Autodesk Inventor part; units mm, degrees
(part 3 of 4)
  spline S550 degree 2 poles (-51.993, -43.6703) (-51.7908, -43.577) (-51.241, -43.5069) (-50.922, -43.4888) knots 0 0 0 1 2 2 2
  line L465 (-50.922, -43.4888) -> (-50.922, -43.411)
  spline S551 degree 2 poles (-50.922, -43.411) (-50.922, -43.271) (-51.0076, -43.0972) (-51.0854, -43.0479) knots 0 0 0 1 2 2 2
  spline S552 degree 2 poles (-51.0854, -43.0479) (-51.1632, -42.9987) (-51.3862, -42.9676) (-51.5055, -42.9676) knots 0 0 0 1 2 2 2
  spline S553 degree 2 poles (-51.5055, -42.9676) (-51.6455, -42.9676) (-52.0241, -43.0505) (-52.2135, -43.1309) knots 0 0 0 1 2 2 2
  line L466 (-52.2135, -43.1309) -> (-52.2368, -43.1309)
  line L467 (-52.2368, -43.1309) -> (-52.2368, -42.7186)
  spline S554 degree 2 poles (-52.2368, -42.7186) (-52.1253, -42.6875) (-51.7078, -42.6097) (-51.5029, -42.6097) knots 0 0 0 1 2 2 2
  spline S555 degree 2 poles (-51.5029, -42.6097) (-51.254, -42.6097) (-50.9143, -42.6875) (-50.7794, -42.7886) knots 0 0 0 1 2 2 2
  spline S556 degree 2 poles (-50.7794, -42.7886) (-50.6472, -42.8872) (-50.5175, -43.2009) (-50.5175, -43.4266) knots 0 0 0 1 2 2 2
  line L468 (-50.5175, -43.4266) -> (-50.5175, -45.068)
  line L469 (-50.5175, -45.068) -> (-50.922, -45.068)
  line L470 (-50.922, -45.068) -> (-50.922, -44.8139)
  line L471 (-50.922, -44.4768) -> (-50.922, -43.8103)
  spline S557 degree 2 poles (-50.922, -43.8103) (-51.0673, -43.8233) (-51.5055, -43.8674) (-51.643, -43.9089) knots 0 0 0 1 2 2 2
  spline S558 degree 2 poles (-51.643, -43.9089) (-51.8037, -43.9582) (-52.0138, -44.163) (-52.0138, -44.3445) knots 0 0 0 1 2 2 2
  spline S559 degree 2 poles (-52.0138, -44.3445) (-52.0138, -44.552) (-51.7804, -44.762) (-51.5574, -44.762) knots 0 0 0 1 2 2 2
  spline S560 degree 2 poles (-51.5574, -44.762) (-51.3681, -44.762) (-51.0569, -44.5987) (-50.922, -44.4768) knots 0 0 0 1 2 2 2
  line L472 (-48.0643, -42.6667) -> (-49.3558, -45.9523)
  line L473 (-49.3558, -45.9523) -> (-49.7888, -45.9523)
  line L474 (-49.7888, -45.9523) -> (-49.3583, -44.9513)
  line L475 (-49.3583, -44.9513) -> (-50.2297, -42.6667)
  line L476 (-50.2297, -42.6667) -> (-49.794, -42.6667)
  line L477 (-49.794, -42.6667) -> (-49.1379, -44.4457)
  line L478 (-49.1379, -44.4457) -> (-48.4844, -42.6667)
  line L479 (-48.4844, -42.6667) -> (-48.0643, -42.6667)
  spline S561 degree 2 poles (-45.7849, -43.8674) (-45.7849, -44.4742) (-46.3684, -45.1355) (-46.8559, -45.1355) knots 0 0 0 1 2 2 2
  spline S562 degree 2 poles (-46.8559, -45.1355) (-47.3564, -45.1355) (-47.9295, -44.4535) (-47.9295, -43.8674) knots 0 0 0 1 2 2 2
  spline S563 degree 2 poles (-47.9295, -43.8674) (-47.9295, -43.2658) (-47.3383, -42.5993) (-46.8559, -42.5993) knots 0 0 0 1 2 2 2
  spline S564 degree 2 poles (-46.8559, -42.5993) (-46.3684, -42.5993) (-45.7849, -43.2632) (-45.7849, -43.8674) knots 0 0 0 1 2 2 2
  spline S565 degree 2 poles (-46.2024, -43.8674) (-46.2024, -43.4006) (-46.5421, -42.9468) (-46.8559, -42.9468) knots 0 0 0 1 2 2 2
  spline S566 degree 2 poles (-46.8559, -42.9468) (-47.1697, -42.9468) (-47.512, -43.4006) (-47.512, -43.8674) knots 0 0 0 1 2 2 2
  spline S567 degree 2 poles (-47.512, -43.8674) (-47.512, -44.3212) (-47.1697, -44.788) (-46.8559, -44.788) knots 0 0 0 1 2 2 2
  spline S568 degree 2 poles (-46.8559, -44.788) (-46.5447, -44.788) (-46.2024, -44.329) (-46.2024, -43.8674) knots 0 0 0 1 2 2 2
  line L480 (-42.4605, -42.6667) -> (-43.0699, -45.068)
  line L481 (-43.0699, -45.068) -> (-43.4433, -45.068)
  line L482 (-43.4433, -45.068) -> (-44.0293, -43.2165)
  line L483 (-44.0293, -43.2165) -> (-44.6128, -45.068)
  line L484 (-44.6128, -45.068) -> (-44.9836, -45.068)
  line L485 (-44.9836, -45.068) -> (-45.5982, -42.6667)
  line L486 (-45.5982, -42.6667) -> (-45.1781, -42.6667)
  line L487 (-45.1781, -42.6667) -> (-44.7528, -44.5261)
  line L488 (-44.7528, -44.5261) -> (-44.1849, -42.6667)
  line L489 (-44.1849, -42.6667) -> (-43.8504, -42.6667)
  line L490 (-43.8504, -42.6667) -> (-43.2669, -44.5261)
  line L491 (-43.2669, -44.5261) -> (-42.8676, -42.6667)
  line L492 (-42.8676, -42.6667) -> (-42.4605, -42.6667)
  spline S569 degree 2 poles (-40.7671, -44.8139) (-40.8164, -44.8502) (-40.9823, -44.9799) (-41.0601, -45.0188) knots 0 0 0 1 2 2 2
  spline S570 degree 2 poles (-41.0601, -45.0188) (-41.1665, -45.0758) (-41.3661, -45.1355) (-41.5477, -45.1355) knots 0 0 0 1 2 2 2
  spline S571 degree 2 poles (-41.5477, -45.1355) (-41.6955, -45.1355) (-41.9626, -45.024) (-42.0637, -44.9228) knots 0 0 0 1 2 2 2
  spline S572 degree 2 poles (-42.0637, -44.9228) (-42.1596, -44.8243) (-42.2763, -44.5338) (-42.2763, -44.3731) knots 0 0 0 1 2 2 2
  spline S573 degree 2 poles (-42.2763, -44.3731) (-42.2763, -44.1241) (-42.0663, -43.7714) (-41.8381, -43.6703) knots 0 0 0 1 2 2 2
  spline S574 degree 2 poles (-41.8381, -43.6703) (-41.6358, -43.577) (-41.0861, -43.5069) (-40.7671, -43.4888) knots 0 0 0 1 2 2 2
  line L493 (-40.7671, -43.4888) -> (-40.7671, -43.411)
  spline S575 degree 2 poles (-40.7671, -43.411) (-40.7671, -43.271) (-40.8527, -43.0972) (-40.9305, -43.0479) knots 0 0 0 1 2 2 2
  spline S576 degree 2 poles (-40.9305, -43.0479) (-41.0083, -42.9987) (-41.2313, -42.9676) (-41.3506, -42.9676) knots 0 0 0 1 2 2 2
  spline S577 degree 2 poles (-41.3506, -42.9676) (-41.4906, -42.9676) (-41.8692, -43.0505) (-42.0585, -43.1309) knots 0 0 0 1 2 2 2
  line L494 (-42.0585, -43.1309) -> (-42.0818, -43.1309)
  line L495 (-42.0818, -43.1309) -> (-42.0818, -42.7186)
  spline S578 degree 2 poles (-42.0818, -42.7186) (-41.9703, -42.6875) (-41.5528, -42.6097) (-41.348, -42.6097) knots 0 0 0 1 2 2 2
  spline S579 degree 2 poles (-41.348, -42.6097) (-41.099, -42.6097) (-40.7593, -42.6875) (-40.6245, -42.7886) knots 0 0 0 1 2 2 2
  spline S580 degree 2 poles (-40.6245, -42.7886) (-40.4922, -42.8872) (-40.3626, -43.2009) (-40.3626, -43.4266) knots 0 0 0 1 2 2 2
  line L496 (-40.3626, -43.4266) -> (-40.3626, -45.068)
  line L497 (-40.3626, -45.068) -> (-40.7671, -45.068)
  line L498 (-40.7671, -45.068) -> (-40.7671, -44.8139)
  line L499 (-40.7671, -44.4768) -> (-40.7671, -43.8103)
  spline S581 degree 2 poles (-40.7671, -43.8103) (-40.9123, -43.8233) (-41.3506, -43.8674) (-41.488, -43.9089) knots 0 0 0 1 2 2 2
  spline S582 degree 2 poles (-41.488, -43.9089) (-41.6488, -43.9582) (-41.8588, -44.163) (-41.8588, -44.3445) knots 0 0 0 1 2 2 2
  spline S583 degree 2 poles (-41.8588, -44.3445) (-41.8588, -44.552) (-41.6254, -44.762) (-41.4024, -44.762) knots 0 0 0 1 2 2 2
  spline S584 degree 2 poles (-41.4024, -44.762) (-41.2131, -44.762) (-40.9019, -44.5987) (-40.7671, -44.4768) knots 0 0 0 1 2 2 2
  spline S585 degree 2 poles (-95.7083, -4.693) (-95.7083, -4.8875) (-95.842, -5.2327) (-95.9757, -5.3543) knots 0 0 0 1 2 2 2
  spline S586 degree 2 poles (-95.9757, -5.3543) (-96.1264, -5.4904) (-96.5373, -5.6193) (-96.8047, -5.6193) knots 0 0 0 1 2 2 2
  spline S587 degree 2 poles (-96.8047, -5.6193) (-97.0041, -5.6193) (-97.3541, -5.5901) (-97.4878, -5.5609) knots 0 0 0 1 2 2 2
  line L500 (-97.4878, -5.5609) -> (-97.4878, -4.9531)
  line L501 (-97.4878, -4.9531) -> (-97.4198, -4.9531)
  spline S588 degree 2 poles (-97.4198, -4.9531) (-97.3298, -4.9896) (-97.1329, -5.0528) (-96.9773, -5.0528) knots 0 0 0 1 2 2 2
  spline S589 degree 2 poles (-96.9773, -5.0528) (-96.778, -5.0528) (-96.5616, -4.941) (-96.5178, -4.8389) knots 0 0 0 1 2 2 2
  spline S590 degree 2 poles (-96.5178, -4.8389) (-96.4716, -4.7392) (-96.4619, -4.4815) (-96.4619, -4.321) knots 0 0 0 1 2 2 2
  line L502 (-96.4619, -4.321) -> (-96.4619, -3.1176)
  line L503 (-96.4619, -3.1176) -> (-97.1475, -3.1176)
  line L504 (-97.1475, -3.1176) -> (-97.1475, -2.5731)
  line L505 (-97.1475, -2.5731) -> (-95.7083, -2.5731)
  line L506 (-95.7083, -2.5731) -> (-95.7083, -4.693)
  spline S591 degree 2 poles (-93.0024, -4.6638) (-93.0024, -4.8851) (-93.1653, -5.2473) (-93.3233, -5.3737) knots 0 0 0 1 2 2 2
  spline S592 degree 2 poles (-93.3233, -5.3737) (-93.4814, -5.5001) (-93.9117, -5.6363) (-94.2204, -5.6363) knots 0 0 0 1 2 2 2
  spline S593 degree 2 poles (-94.2204, -5.6363) (-94.5705, -5.6363) (-95.0713, -5.5196) (-95.2293, -5.4466) knots 0 0 0 1 2 2 2
  line L507 (-95.2293, -5.4466) -> (-95.2293, -4.7951)
  line L508 (-95.2293, -4.7951) -> (-95.1564, -4.7951)
  spline S594 degree 2 poles (-95.1564, -4.7951) (-94.9911, -4.8996) (-94.5462, -5.0552) (-94.3614, -5.0552) knots 0 0 0 1 2 2 2
  spline S595 degree 2 poles (-94.3614, -5.0552) (-94.252, -5.0552) (-93.9968, -5.0163) (-93.9092, -4.9531) knots 0 0 0 1 2 2 2
  spline S596 degree 2 poles (-93.9092, -4.9531) (-93.8412, -4.9021) (-93.7585, -4.7538) (-93.7585, -4.6201) knots 0 0 0 1 2 2 2
  spline S597 degree 2 poles (-93.7585, -4.6201) (-93.7585, -4.4864) (-93.8752, -4.3429) (-93.9724, -4.3089) knots 0 0 0 1 2 2 2
  spline S598 degree 2 poles (-93.9724, -4.3089) (-94.0697, -4.2749) (-94.3395, -4.2676) (-94.4441, -4.2676) knots 0 0 0 1 2 2 2
  line L509 (-94.4441, -4.2676) -> (-94.5729, -4.2676)
  line L510 (-94.5729, -4.2676) -> (-94.5729, -3.74)
  line L511 (-94.5729, -3.74) -> (-94.4538, -3.74)
  spline S599 degree 2 poles (-94.4538, -3.74) (-94.3177, -3.74) (-94.0867, -3.7157) (-94.0065, -3.6792) knots 0 0 0 1 2 2 2
  spline S600 degree 2 poles (-94.0065, -3.6792) (-93.9263, -3.6403) (-93.8363, -3.5042) (-93.8363, -3.3875) knots 0 0 0 1 2 2 2
  spline S601 degree 2 poles (-93.8363, -3.3875) (-93.8363, -3.2951) (-93.9214, -3.1808) (-93.9822, -3.1492) knots 0 0 0 1 2 2 2
  spline S602 degree 2 poles (-93.9822, -3.1492) (-94.0551, -3.1128) (-94.2496, -3.0885) (-94.3177, -3.0885) knots 0 0 0 1 2 2 2
  spline S603 degree 2 poles (-94.3177, -3.0885) (-94.4271, -3.0885) (-94.658, -3.1395) (-94.765, -3.1808) knots 0 0 0 1 2 2 2
  spline S604 degree 2 poles (-94.765, -3.1808) (-94.8501, -3.2125) (-95.0348, -3.3146) (-95.0786, -3.3413) knots 0 0 0 1 2 2 2
  line L512 (-95.0786, -3.3413) -> (-95.1418, -3.3413)
  line L513 (-95.1418, -3.3413) -> (-95.1418, -2.6995)
  spline S605 degree 2 poles (-95.1418, -2.6995) (-94.9862, -2.6338) (-94.4611, -2.5099) (-94.1864, -2.5099) knots 0 0 0 1 2 2 2
  spline S606 degree 2 poles (-94.1864, -2.5099) (-93.919, -2.5099) (-93.5251, -2.6022) (-93.3865, -2.6922) knots 0 0 0 1 2 2 2
  spline S607 degree 2 poles (-93.3865, -2.6922) (-93.2334, -2.787) (-93.0802, -3.0787) (-93.0802, -3.2611) knots 0 0 0 1 2 2 2
  spline S608 degree 2 poles (-93.0802, -3.2611) (-93.0802, -3.5188) (-93.3768, -3.9029) (-93.6199, -3.9588) knots 0 0 0 1 2 2 2
  line L514 (-93.6199, -3.9588) -> (-93.6199, -3.988)
  spline S609 degree 2 poles (-93.6199, -3.988) (-93.513, -4.0026) (-93.3088, -4.0804) (-93.2115, -4.1679) knots 0 0 0 1 2 2 2
  spline S610 degree 2 poles (-93.2115, -4.1679) (-93.1216, -4.2457) (-93.0024, -4.4937) (-93.0024, -4.6638) knots 0 0 0 1 2 2 2
  spline S611 degree 2 poles (-90.316, -4.552) (-90.316, -5.0261) (-90.9165, -5.6363) (-91.4417, -5.6363) knots 0 0 0 1 2 2 2
  spline S612 degree 2 poles (-91.4417, -5.6363) (-91.7042, -5.6363) (-92.1151, -5.4855) (-92.2585, -5.3372) knots 0 0 0 1 2 2 2
  spline S613 degree 2 poles (-92.2585, -5.3372) (-92.4287, -5.1646) (-92.611, -4.6176) (-92.611, -4.236) knots 0 0 0 1 2 2 2
  spline S614 degree 2 poles (-92.611, -4.236) (-92.611, -3.8421) (-92.4408, -3.2295) (-92.2488, -2.9937) knots 0 0 0 1 2 2 2
  spline S615 degree 2 poles (-92.2488, -2.9937) (-92.0665, -2.77) (-91.4733, -2.5172) (-91.0673, -2.5172) knots 0 0 0 1 2 2 2
  spline S616 degree 2 poles (-91.0673, -2.5172) (-90.919, -2.5172) (-90.6224, -2.5561) (-90.5689, -2.5682) knots 0 0 0 1 2 2 2
  line L515 (-90.5689, -2.5682) -> (-90.5689, -3.1565)
  line L516 (-90.5689, -3.1565) -> (-90.6224, -3.1565)
  spline S617 degree 2 poles (-90.6224, -3.1565) (-90.6759, -3.1298) (-90.919, -3.0642) (-91.0746, -3.0642) knots 0 0 0 1 2 2 2
  spline S618 degree 2 poles (-91.0746, -3.0642) (-91.4271, -3.0642) (-91.8112, -3.4361) (-91.8574, -3.7813) knots 0 0 0 1 2 2 2
  spline S619 degree 2 poles (-91.8574, -3.7813) (-91.7091, -3.6865) (-91.4052, -3.5747) (-91.2131, -3.5747) knots 0 0 0 1 2 2 2
  spline S620 degree 2 poles (-91.2131, -3.5747) (-91.0502, -3.5747) (-90.7658, -3.6622) (-90.6564, -3.7449) knots 0 0 0 1 2 2 2
  spline S621 degree 2 poles (-90.6564, -3.7449) (-90.5008, -3.864) (-90.316, -4.2505) (-90.316, -4.552) knots 0 0 0 1 2 2 2
  spline S622 degree 2 poles (-91.1937, -5.0042) (-91.1353, -4.9313) (-91.0721, -4.7611) (-91.0721, -4.5885) knots 0 0 0 1 2 2 2
  spline S623 degree 2 poles (-91.0721, -4.5885) (-91.0721, -4.4426) (-91.1451, -4.253) (-91.2107, -4.1971) knots 0 0 0 1 2 2 2
  spline S624 degree 2 poles (-91.2107, -4.1971) (-91.2788, -4.1387) (-91.4465, -4.0974) (-91.5413, -4.0974) knots 0 0 0 1 2 2 2
  spline S625 degree 2 poles (-91.5413, -4.0974) (-91.6216, -4.0974) (-91.7869, -4.1387) (-91.8598, -4.1679) knots 0 0 0 1 2 2 2
  spline S626 degree 2 poles (-91.8598, -4.1679) (-91.8598, -4.1873) (-91.8647, -4.2797) (-91.8647, -4.3502) knots 0 0 0 1 2 2 2
  spline S627 degree 2 poles (-91.8647, -4.3502) (-91.8647, -4.6103) (-91.7747, -4.924) (-91.7042, -5.0042) knots 0 0 0 1 2 2 2
  spline S628 degree 2 poles (-91.7042, -5.0042) (-91.6532, -5.0698) (-91.517, -5.1257) (-91.4441, -5.1257) knots 0 0 0 1 2 2 2
  spline S629 degree 2 poles (-91.4441, -5.1257) (-91.3833, -5.1257) (-91.2423, -5.065) (-91.1937, -5.0042) knots 0 0 0 1 2 2 2
  spline S630 degree 2 poles (-87.6783, -4.7392) (-87.6783, -4.9313) (-87.8387, -5.2643) (-87.9919, -5.3859) knots 0 0 0 1 2 2 2
  spline S631 degree 2 poles (-87.9919, -5.3859) (-88.1451, -5.5074) (-88.5851, -5.6436) (-88.8695, -5.6436) knots 0 0 0 1 2 2 2
  spline S632 degree 2 poles (-88.8695, -5.6436) (-89.1734, -5.6436) (-89.628, -5.505) (-89.7739, -5.3859) knots 0 0 0 1 2 2 2
  spline S633 degree 2 poles (-89.7739, -5.3859) (-89.9173, -5.2667) (-90.0535, -4.9434) (-90.0535, -4.7635) knots 0 0 0 1 2 2 2
  spline S634 degree 2 poles (-90.0535, -4.7635) (-90.0535, -4.5058) (-89.769, -4.163) (-89.4992, -4.0488) knots 0 0 0 1 2 2 2
  line L517 (-89.4992, -4.0488) -> (-89.4992, -4.0366)
  spline S635 degree 2 poles (-89.4992, -4.0366) (-89.7642, -3.9078) (-89.9733, -3.5407) (-89.9733, -3.3146) knots 0 0 0 1 2 2 2
  spline S636 degree 2 poles (-89.9733, -3.3146) (-89.9733, -3.1492) (-89.8274, -2.8599) (-89.684, -2.7457) knots 0 0 0 1 2 2 2
  spline S637 degree 2 poles (-89.684, -2.7457) (-89.5454, -2.6363) (-89.1248, -2.505) (-88.8622, -2.505) knots 0 0 0 1 2 2 2
  spline S638 degree 2 poles (-88.8622, -2.505) (-88.5851, -2.505) (-88.1718, -2.6241) (-88.0381, -2.7214) knots 0 0 0 1 2 2 2
  spline S639 degree 2 poles (-88.0381, -2.7214) (-87.9019, -2.8186) (-87.7561, -3.1006) (-87.7561, -3.2635) knots 0 0 0 1 2 2 2
  spline S640 degree 2 poles (-87.7561, -3.2635) (-87.7561, -3.4774) (-88.0041, -3.8202) (-88.2593, -3.9394) knots 0 0 0 1 2 2 2
  line L518 (-88.2593, -3.9394) -> (-88.2593, -3.9491)
  spline S641 degree 2 poles (-88.2593, -3.9491) (-87.9603, -4.0706) (-87.6783, -4.4645) (-87.6783, -4.7392) knots 0 0 0 1 2 2 2
  spline S642 degree 2 poles (-88.4222, -4.7708) (-88.4222, -4.6225) (-88.5486, -4.4669) (-88.7528, -4.3672) knots 0 0 0 1 2 2 2
  spline S643 degree 2 poles (-88.7528, -4.3672) (-88.8112, -4.3405) (-89.0324, -4.2554) (-89.1175, -4.2189) knots 0 0 0 1 2 2 2
  spline S644 degree 2 poles (-89.1175, -4.2189) (-89.1953, -4.2967) (-89.3193, -4.5301) (-89.3193, -4.6687) knots 0 0 0 1 2 2 2
  spline S645 degree 2 poles (-89.3193, -4.6687) (-89.3193, -4.8778) (-89.0519, -5.1282) (-88.8355, -5.1282) knots 0 0 0 1 2 2 2
  spline S646 degree 2 poles (-88.8355, -5.1282) (-88.7747, -5.1282) (-88.624, -5.0893) (-88.5656, -5.0504) knots 0 0 0 1 2 2 2
  spline S647 degree 2 poles (-88.5656, -5.0504) (-88.5, -5.0042) (-88.4222, -4.8778) (-88.4222, -4.7708) knots 0 0 0 1 2 2 2
  spline S648 degree 2 poles (-88.4878, -3.351) (-88.4878, -3.1979) (-88.6896, -3.0155) (-88.8622, -3.0155) knots 0 0 0 1 2 2 2
  spline S649 degree 2 poles (-88.8622, -3.0155) (-89.0276, -3.0155) (-89.2293, -3.1808) (-89.2293, -3.3024) knots 0 0 0 1 2 2 2
  spline S650 degree 2 poles (-89.2293, -3.3024) (-89.2293, -3.4215) (-89.1078, -3.5698) (-88.9789, -3.6306) knots 0 0 0 1 2 2 2
  spline S651 degree 2 poles (-88.9789, -3.6306) (-88.923, -3.6598) (-88.7674, -3.7206) (-88.6386, -3.7692) knots 0 0 0 1 2 2 2
  spline S652 degree 2 poles (-88.6386, -3.7692) (-88.5608, -3.6671) (-88.4878, -3.475) (-88.4878, -3.351) knots 0 0 0 1 2 2 2
  line L519 (-86.4457, -5.5731) -> (-87.158, -5.5731)
  line L520 (-87.158, -5.5731) -> (-87.158, -4.7805)
  line L521 (-87.158, -4.7805) -> (-86.4457, -4.7805)
  line L522 (-86.4457, -4.7805) -> (-86.4457, -5.5731)
  line L523 (-86.4457, -4.1022) -> (-87.158, -4.1022)
  line L524 (-87.158, -4.1022) -> (-87.158, -3.3097)
  line L525 (-87.158, -3.3097) -> (-86.4457, -3.3097)
  line L526 (-86.4457, -3.3097) -> (-86.4457, -4.1022)
  line L527 (-84.8582, -5.5731) -> (-83.8444, -2.5731)
  line L528 (-83.8444, -2.5731) -> (-83.0227, -2.5731)
  line L529 (-83.0227, -2.5731) -> (-82.0089, -5.5731)
  line L530 (-82.0089, -5.5731) -> (-82.7844, -5.5731)
  line L531 (-82.7844, -5.5731) -> (-82.9716, -4.9604)
  line L532 (-82.9716, -4.9604) -> (-83.9149, -4.9604)
  line L533 (-83.9149, -4.9604) -> (-84.1045, -5.5731)
  line L534 (-84.1045, -5.5731) -> (-84.8582, -5.5731)
  line L535 (-83.137, -4.4159) -> (-83.4433, -3.424)
  line L536 (-83.4433, -3.424) -> (-83.752, -4.4159)
  line L537 (-83.752, -4.4159) -> (-83.137, -4.4159)
  spline S653 degree 2 poles (-79.0332, -4.0755) (-79.0332, -4.4961) (-79.4003, -5.1573) (-79.6799, -5.3348) knots 0 0 0 1 2 2 2
  spline S654 degree 2 poles (-79.6799, -5.3348) (-79.9133, -5.4855) (-80.4627, -5.5731) (-80.7715, -5.5731) knots 0 0 0 1 2 2 2
  line L538 (-80.7715, -5.5731) -> (-81.7099, -5.5731)
  line L539 (-81.7099, -5.5731) -> (-81.7099, -2.5731)
  line L540 (-81.7099, -2.5731) -> (-80.7812, -2.5731)
  spline S655 degree 2 poles (-80.7812, -2.5731) (-80.4652, -2.5731) (-79.9133, -2.6533) (-79.6702, -2.8089) knots 0 0 0 1 2 2 2
  spline S656 degree 2 poles (-79.6702, -2.8089) (-79.376, -2.9985) (-79.0332, -3.6403) (-79.0332, -4.0755) knots 0 0 0 1 2 2 2
  spline S657 degree 2 poles (-79.8063, -4.0706) (-79.8063, -3.774) (-80.0105, -3.351) (-80.2196, -3.2319) knots 0 0 0 1 2 2 2
  spline S658 degree 2 poles (-80.2196, -3.2319) (-80.3728, -3.1492) (-80.7083, -3.1322) (-80.9417, -3.1322) knots 0 0 0 1 2 2 2
  line L541 (-80.9417, -3.1322) -> (-80.9562, -3.1322)
  line L542 (-80.9562, -3.1322) -> (-80.9562, -5.0115)
  line L543 (-80.9562, -5.0115) -> (-80.9417, -5.0115)
  spline S659 degree 2 poles (-80.9417, -5.0115) (-80.6888, -5.0115) (-80.3412, -4.9945) (-80.1831, -4.8948) knots 0 0 0 1 2 2 2
  spline S660 degree 2 poles (-80.1831, -4.8948) (-79.9984, -4.7781) (-79.8063, -4.3672) (-79.8063, -4.0706) knots 0 0 0 1 2 2 2
  line L544 (-76.0818, -2.5731) -> (-77.1126, -5.5731)
  line L545 (-77.1126, -5.5731) -> (-77.8979, -5.5731)
  line L546 (-77.8979, -5.5731) -> (-78.9287, -2.5731)
  line L547 (-78.9287, -2.5731) -> (-78.1483, -2.5731)
  line L548 (-78.1483, -2.5731) -> (-77.4943, -4.6079)
  line L549 (-77.4943, -4.6079) -> (-76.8428, -2.5731)
  line L550 (-76.8428, -2.5731) -> (-76.0818, -2.5731)
  line L551 (-76.1256, -5.5731) -> (-75.1118, -2.5731)
  line L552 (-75.1118, -2.5731) -> (-74.2901, -2.5731)
  line L553 (-74.2901, -2.5731) -> (-73.2763, -5.5731)
  line L554 (-73.2763, -5.5731) -> (-74.0519, -5.5731)
  line L555 (-74.0519, -5.5731) -> (-74.2391, -4.9604)
  line L556 (-74.2391, -4.9604) -> (-75.1823, -4.9604)
  line L557 (-75.1823, -4.9604) -> (-75.372, -5.5731)
  line L558 (-75.372, -5.5731) -> (-76.1256, -5.5731)
  line L559 (-74.4044, -4.4159) -> (-74.7107, -3.424)
  line L560 (-74.7107, -3.424) -> (-75.0194, -4.4159)
  line L561 (-75.0194, -4.4159) -> (-74.4044, -4.4159)
  line L562 (-70.4076, -5.5731) -> (-71.1321, -5.5731)
  line L563 (-71.1321, -5.5731) -> (-72.2893, -3.4823)
  line L564 (-72.2893, -3.4823) -> (-72.2893, -5.5731)
  line L565 (-72.2893, -5.5731) -> (-72.9773, -5.5731)
  line L566 (-72.9773, -5.5731) -> (-72.9773, -2.5731)
  line L567 (-72.9773, -2.5731) -> (-72.0535, -2.5731)
  line L568 (-72.0535, -2.5731) -> (-71.0956, -4.2919)
  line L569 (-71.0956, -4.2919) -> (-71.0956, -2.5731)
  line L570 (-71.0956, -2.5731) -> (-70.4076, -2.5731)
  line L571 (-70.4076, -2.5731) -> (-70.4076, -5.5731)
  spline S661 degree 2 poles (-68.5041, -5.6314) (-69.1799, -5.6314) (-69.9724, -4.8146) (-69.9724, -4.0755) knots 0 0 0 1 2 2 2
  spline S662 degree 2 poles (-69.9724, -4.0755) (-69.9724, -3.3632) (-69.1775, -2.5147) (-68.5016, -2.5147) knots 0 0 0 1 2 2 2
  spline S663 degree 2 poles (-68.5016, -2.5147) (-68.3241, -2.5147) (-68.0373, -2.5561) (-67.906, -2.5901) knots 0 0 0 1 2 2 2
  spline S664 degree 2 poles (-67.906, -2.5901) (-67.8039, -2.6217) (-67.5632, -2.7262) (-67.4878, -2.7651) knots 0 0 0 1 2 2 2
  line L572 (-67.4878, -2.7651) -> (-67.4878, -3.4799)
  line L573 (-67.4878, -3.4799) -> (-67.5632, -3.4799)
  spline S665 degree 2 poles (-67.5632, -3.4799) (-67.6191, -3.4313) (-67.7844, -3.2951) (-67.889, -3.2319) knots 0 0 0 1 2 2 2
  spline S666 degree 2 poles (-67.889, -3.2319) (-67.9935, -3.1663) (-68.2439, -3.0763) (-68.3825, -3.0763) knots 0 0 0 1 2 2 2
  spline S667 degree 2 poles (-68.3825, -3.0763) (-68.5454, -3.0763) (-68.8152, -3.1784) (-68.9392, -3.3073) knots 0 0 0 1 2 2 2
  spline S668 degree 2 poles (-68.9392, -3.3073) (-69.0511, -3.4215) (-69.1945, -3.8129) (-69.1945, -4.0779) knots 0 0 0 1 2 2 2
  spline S669 degree 2 poles (-69.1945, -4.0779) (-69.1945, -4.3575) (-69.0462, -4.7392) (-68.9246, -4.8559) knots 0 0 0 1 2 2 2
  spline S670 degree 2 poles (-68.9246, -4.8559) (-68.8079, -4.9702) (-68.5211, -5.0698) (-68.3776, -5.0698) knots 0 0 0 1 2 2 2
  spline S671 degree 2 poles (-68.3776, -5.0698) (-68.2293, -5.0698) (-67.9595, -4.9702) (-67.8671, -4.9094) knots 0 0 0 1 2 2 2
  spline S672 degree 2 poles (-67.8671, -4.9094) (-67.765, -4.8486) (-67.6118, -4.7197) (-67.5559, -4.6687) knots 0 0 0 1 2 2 2
  line L574 (-67.5559, -4.6687) -> (-67.4878, -4.6687)
  line L575 (-67.4878, -4.6687) -> (-67.4878, -5.3737)
  spline S673 degree 2 poles (-67.4878, -5.3737) (-67.5705, -5.4126) (-67.7869, -5.5099) (-67.9036, -5.5439) knots 0 0 0 1 2 2 2
  spline S674 degree 2 poles (-67.9036, -5.5439) (-68.0446, -5.5877) (-68.2901, -5.6314) (-68.5041, -5.6314) knots 0 0 0 1 2 2 2
  line L576 (-67.0429, -5.5731) -> (-67.0429, -2.5731)
  line L577 (-67.0429, -2.5731) -> (-65.0154, -2.5731)
  line L578 (-65.0154, -2.5731) -> (-65.0154, -3.1444)
  line L579 (-65.0154, -3.1444) -> (-66.2942, -3.1444)
  line L580 (-66.2942, -3.1444) -> (-66.2942, -3.6719)
  line L581 (-66.2942, -3.6719) -> (-65.1151, -3.6719)
  line L582 (-65.1151, -3.6719) -> (-65.1151, -4.2432)
  line L583 (-65.1151, -4.2432) -> (-66.2942, -4.2432)
  line L584 (-66.2942, -4.2432) -> (-66.2942, -5.0018)
  line L585 (-66.2942, -5.0018) -> (-65.0154, -5.0018)
  line L586 (-65.0154, -5.0018) -> (-65.0154, -5.5731)
  line L587 (-65.0154, -5.5731) -> (-67.0429, -5.5731)
  spline S675 degree 2 poles (-61.8282, -4.0755) (-61.8282, -4.4961) (-62.1953, -5.1573) (-62.4749, -5.3348) knots 0 0 0 1 2 2 2
  spline S676 degree 2 poles (-62.4749, -5.3348) (-62.7083, -5.4855) (-63.2577, -5.5731) (-63.5664, -5.5731) knots 0 0 0 1 2 2 2
  line L588 (-63.5664, -5.5731) -> (-64.5049, -5.5731)
  line L589 (-64.5049, -5.5731) -> (-64.5049, -2.5731)
  line L590 (-64.5049, -2.5731) -> (-63.5762, -2.5731)
  spline S677 degree 2 poles (-63.5762, -2.5731) (-63.2601, -2.5731) (-62.7083, -2.6533) (-62.4652, -2.8089) knots 0 0 0 1 2 2 2
  spline S678 degree 2 poles (-62.4652, -2.8089) (-62.171, -2.9985) (-61.8282, -3.6403) (-61.8282, -4.0755) knots 0 0 0 1 2 2 2
  spline S679 degree 2 poles (-62.6013, -4.0706) (-62.6013, -3.774) (-62.8055, -3.351) (-63.0146, -3.2319) knots 0 0 0 1 2 2 2
  spline S680 degree 2 poles (-63.0146, -3.2319) (-63.1677, -3.1492) (-63.5032, -3.1322) (-63.7366, -3.1322) knots 0 0 0 1 2 2 2
  line L591 (-63.7366, -3.1322) -> (-63.7512, -3.1322)
  line L592 (-63.7512, -3.1322) -> (-63.7512, -5.0115)
  line L593 (-63.7512, -5.0115) -> (-63.7366, -5.0115)
  spline S681 degree 2 poles (-63.7366, -5.0115) (-63.4838, -5.0115) (-63.1361, -4.9945) (-62.9781, -4.8948) knots 0 0 0 1 2 2 2
  spline S682 degree 2 poles (-62.9781, -4.8948) (-62.7934, -4.7781) (-62.6013, -4.3672) (-62.6013, -4.0706) knots 0 0 0 1 2 2 2
  spline S683 degree 2 poles (-57.4959, -4.0755) (-57.4959, -4.4961) (-57.863, -5.1573) (-58.1426, -5.3348) knots 0 0 0 1 2 2 2
  spline S684 degree 2 poles (-58.1426, -5.3348) (-58.376, -5.4855) (-58.9254, -5.5731) (-59.2342, -5.5731) knots 0 0 0 1 2 2 2
  line L594 (-59.2342, -5.5731) -> (-60.1726, -5.5731)
  line L595 (-60.1726, -5.5731) -> (-60.1726, -2.5731)
  line L596 (-60.1726, -2.5731) -> (-59.2439, -2.5731)
  spline S685 degree 2 poles (-59.2439, -2.5731) (-58.9279, -2.5731) (-58.376, -2.6533) (-58.1329, -2.8089) knots 0 0 0 1 2 2 2
  spline S686 degree 2 poles (-58.1329, -2.8089) (-57.8387, -2.9985) (-57.4959, -3.6403) (-57.4959, -4.0755) knots 0 0 0 1 2 2 2
  spline S687 degree 2 poles (-58.269, -4.0706) (-58.269, -3.774) (-58.4733, -3.351) (-58.6823, -3.2319) knots 0 0 0 1 2 2 2
  spline S688 degree 2 poles (-58.6823, -3.2319) (-58.8355, -3.1492) (-59.171, -3.1322) (-59.4044, -3.1322) knots 0 0 0 1 2 2 2
  line L597 (-59.4044, -3.1322) -> (-59.419, -3.1322)
  line L598 (-59.419, -3.1322) -> (-59.419, -5.0115)
  line L599 (-59.419, -5.0115) -> (-59.4044, -5.0115)
  spline S689 degree 2 poles (-59.4044, -5.0115) (-59.1515, -5.0115) (-58.8039, -4.9945) (-58.6459, -4.8948) knots 0 0 0 1 2 2 2
  spline S690 degree 2 poles (-58.6459, -4.8948) (-58.4611, -4.7781) (-58.269, -4.3672) (-58.269, -4.0706) knots 0 0 0 1 2 2 2
  line L600 (-55.5559, -5.5731) -> (-57.1702, -5.5731)
  line L601 (-57.1702, -5.5731) -> (-57.1702, -5.0504)
  line L602 (-57.1702, -5.0504) -> (-56.7399, -5.0504)
  line L603 (-56.7399, -5.0504) -> (-56.7399, -3.0958)
  line L604 (-56.7399, -3.0958) -> (-57.1702, -3.0958)
  line L605 (-57.1702, -3.0958) -> (-57.1702, -2.5731)
  line L606 (-57.1702, -2.5731) -> (-55.5559, -2.5731)
  line L607 (-55.5559, -2.5731) -> (-55.5559, -3.0958)
  line L608 (-55.5559, -3.0958) -> (-55.9862, -3.0958)
  line L609 (-55.9862, -3.0958) -> (-55.9862, -5.0504)
  line L610 (-55.9862, -5.0504) -> (-55.5559, -5.0504)
  line L611 (-55.5559, -5.0504) -> (-55.5559, -5.5731)
  spline S691 degree 2 poles (-52.748, -3.5188) (-52.748, -3.7278) (-52.8817, -4.1071) (-53.0057, -4.2335) knots 0 0 0 1 2 2 2
  spline S692 degree 2 poles (-53.0057, -4.2335) (-53.081, -4.3137) (-53.2658, -4.445) (-53.3752, -4.4912) knots 0 0 0 1 2 2 2
  spline S693 degree 2 poles (-53.3752, -4.4912) (-53.487, -4.5374) (-53.7472, -4.5909) (-53.9076, -4.5909) knots 0 0 0 1 2 2 2
  line L612 (-53.9076, -4.5909) -> (-54.3015, -4.5909)
  line L613 (-54.3015, -4.5909) -> (-54.3015, -5.5731)
  line L614 (-54.3015, -5.5731) -> (-55.0551, -5.5731)
  line L615 (-55.0551, -5.5731) -> (-55.0551, -2.5731)
  line L616 (-55.0551, -2.5731) -> (-53.8906, -2.5731)
  spline S694 degree 2 poles (-53.8906, -2.5731) (-53.6329, -2.5731) (-53.2561, -2.6679) (-53.1029, -2.77) knots 0 0 0 1 2 2 2
  spline S695 degree 2 poles (-53.1029, -2.77) (-52.9327, -2.8843) (-52.748, -3.2586) (-52.748, -3.5188) knots 0 0 0 1 2 2 2
  spline S696 degree 2 poles (-53.5211, -3.5382) (-53.5211, -3.4094) (-53.6426, -3.227) (-53.7253, -3.193) knots 0 0 0 1 2 2 2
  spline S697 degree 2 poles (-53.7253, -3.193) (-53.8323, -3.1468) (-54.0267, -3.1322) (-54.1945, -3.1322) knots 0 0 0 1 2 2 2
  line L617 (-54.1945, -3.1322) -> (-54.3015, -3.1322)
  line L618 (-54.3015, -3.1322) -> (-54.3015, -4.0317)
  line L619 (-54.3015, -4.0317) -> (-54.248, -4.0317)
  spline S698 degree 2 poles (-54.248, -4.0317) (-54.1434, -4.0317) (-53.9538, -4.0269) (-53.8833, -4.0147) knots 0 0 0 1 2 2 2
  spline S699 degree 2 poles (-53.8833, -4.0147) (-53.8225, -4.005) (-53.6888, -3.9466) (-53.6523, -3.9102) knots 0 0 0 1 2 2 2
  spline S700 degree 2 poles (-53.6523, -3.9102) (-53.5746, -3.8372) (-53.5211, -3.6744) (-53.5211, -3.5382) knots 0 0 0 1 2 2 2
  line L620 (-50.3436, -5.5731) -> (-52.3444, -5.5731)
  line L621 (-52.3444, -5.5731) -> (-52.3444, -2.5731)
  line L622 (-52.3444, -2.5731) -> (-51.5908, -2.5731)
  line L623 (-51.5908, -2.5731) -> (-51.5908, -5.0018)
  line L624 (-51.5908, -5.0018) -> (-50.3436, -5.0018)
  line L625 (-50.3436, -5.0018) -> (-50.3436, -5.5731)
  spline S701 degree 2 poles (-47.2536, -4.0731) (-47.2536, -4.8024) (-48.0316, -5.6363) (-48.7075, -5.6363) knots 0 0 0 1 2 2 2
  spline S702 degree 2 poles (-48.7075, -5.6363) (-49.3857, -5.6363) (-50.1588, -4.7927) (-50.1588, -4.0731) knots 0 0 0 1 2 2 2
  spline S703 degree 2 poles (-50.1588, -4.0731) (-50.1588, -3.351) (-49.3857, -2.5099) (-48.7075, -2.5099) knots 0 0 0 1 2 2 2
  spline S704 degree 2 poles (-48.7075, -2.5099) (-48.0316, -2.5099) (-47.2536, -3.3462) (-47.2536, -4.0731) knots 0 0 0 1 2 2 2
  spline S705 degree 2 poles (-48.0316, -4.0731) (-48.0316, -3.8032) (-48.141, -3.4264) (-48.2358, -3.3073) knots 0 0 0 1 2 2 2
  spline S706 degree 2 poles (-48.2358, -3.3073) (-48.3306, -3.1833) (-48.5737, -3.0763) (-48.705, -3.0763) knots 0 0 0 1 2 2 2
  spline S707 degree 2 poles (-48.705, -3.0763) (-48.8436, -3.0763) (-49.0697, -3.176) (-49.1742, -3.3024) knots 0 0 0 1 2 2 2
  spline S708 degree 2 poles (-49.1742, -3.3024) (-49.2666, -3.4191) (-49.3809, -3.8056) (-49.3809, -4.0731) knots 0 0 0 1 2 2 2
  spline S709 degree 2 poles (-49.3809, -4.0731) (-49.3809, -4.3502) (-49.2715, -4.7149) (-49.1767, -4.8389) knots 0 0 0 1 2 2 2
  spline S710 degree 2 poles (-49.1767, -4.8389) (-49.0818, -4.9629) (-48.8363, -5.0698) (-48.705, -5.0698) knots 0 0 0 1 2 2 2
  spline S711 degree 2 poles (-48.705, -5.0698) (-48.5713, -5.0698) (-48.3233, -4.9556) (-48.2334, -4.834) knots 0 0 0 1 2 2 2
  spline S712 degree 2 poles (-48.2334, -4.834) (-48.1361, -4.7027) (-48.0316, -4.3551) (-48.0316, -4.0731) knots 0 0 0 1 2 2 2
  line L626 (-43.7431, -5.5731) -> (-44.4919, -5.5731)
  line L627 (-44.4919, -5.5731) -> (-44.4919, -3.5844)
  line L628 (-44.4919, -3.5844) -> (-45.0365, -4.868)
  line L629 (-45.0365, -4.868) -> (-45.5519, -4.868)
  line L630 (-45.5519, -4.868) -> (-46.0964, -3.5844)
  line L631 (-46.0964, -3.5844) -> (-46.0964, -5.5731)
  line L632 (-46.0964, -5.5731) -> (-46.8063, -5.5731)
  line L633 (-46.8063, -5.5731) -> (-46.8063, -2.5731)
  line L634 (-46.8063, -2.5731) -> (-45.9384, -2.5731)
  line L635 (-45.9384, -2.5731) -> (-45.2723, -4.0536)
  line L636 (-45.2723, -4.0536) -> (-44.611, -2.5731)
  line L637 (-44.611, -2.5731) -> (-43.7431, -2.5731)
  line L638 (-43.7431, -2.5731) -> (-43.7431, -5.5731)
  line L639 (-43.4441, -5.5731) -> (-42.4303, -2.5731)
  line L640 (-42.4303, -2.5731) -> (-41.6086, -2.5731)
  line L641 (-41.6086, -2.5731) -> (-40.5948, -5.5731)
  line L642 (-40.5948, -5.5731) -> (-41.3703, -5.5731)
  line L643 (-41.3703, -5.5731) -> (-41.5575, -4.9604)
  line L644 (-41.5575, -4.9604) -> (-42.5008, -4.9604)
  line L645 (-42.5008, -4.9604) -> (-42.6904, -5.5731)
  line L646 (-42.6904, -5.5731) -> (-43.4441, -5.5731)
  line L647 (-41.7229, -4.4159) -> (-42.0292, -3.424)
  line L648 (-42.0292, -3.424) -> (-42.3379, -4.4159)
  line L649 (-42.3379, -4.4159) -> (-41.7229, -4.4159)
  spline S713 degree 2 poles (-36.3574, -4.0731) (-36.3574, -4.8024) (-37.1353, -5.6363) (-37.8112, -5.6363) knots 0 0 0 1 2 2 2
  spline S714 degree 2 poles (-37.8112, -5.6363) (-38.4895, -5.6363) (-39.2626, -4.7927) (-39.2626, -4.0731) knots 0 0 0 1 2 2 2
  spline S715 degree 2 poles (-39.2626, -4.0731) (-39.2626, -3.351) (-38.4895, -2.5099) (-37.8112, -2.5099) knots 0 0 0 1 2 2 2
  spline S716 degree 2 poles (-37.8112, -2.5099) (-37.1353, -2.5099) (-36.3574, -3.3462) (-36.3574, -4.0731) knots 0 0 0 1 2 2 2
  spline S717 degree 2 poles (-37.1353, -4.0731) (-37.1353, -3.8032) (-37.2447, -3.4264) (-37.3395, -3.3073) knots 0 0 0 1 2 2 2
  spline S718 degree 2 poles (-37.3395, -3.3073) (-37.4344, -3.1833) (-37.6775, -3.0763) (-37.8087, -3.0763) knots 0 0 0 1 2 2 2
  spline S719 degree 2 poles (-37.8087, -3.0763) (-37.9473, -3.0763) (-38.1734, -3.176) (-38.278, -3.3024) knots 0 0 0 1 2 2 2
  spline S720 degree 2 poles (-38.278, -3.3024) (-38.3703, -3.4191) (-38.4846, -3.8056) (-38.4846, -4.0731) knots 0 0 0 1 2 2 2
  spline S721 degree 2 poles (-38.4846, -4.0731) (-38.4846, -4.3502) (-38.3752, -4.7149) (-38.2804, -4.8389) knots 0 0 0 1 2 2 2
  spline S722 degree 2 poles (-38.2804, -4.8389) (-38.1856, -4.9629) (-37.94, -5.0698) (-37.8087, -5.0698) knots 0 0 0 1 2 2 2
  spline S723 degree 2 poles (-37.8087, -5.0698) (-37.675, -5.0698) (-37.4271, -4.9556) (-37.3371, -4.834) knots 0 0 0 1 2 2 2
  spline S724 degree 2 poles (-37.3371, -4.834) (-37.2399, -4.7027) (-37.1353, -4.3551) (-37.1353, -4.0731) knots 0 0 0 1 2 2 2
  line L650 (-33.9019, -3.1444) -> (-35.1613, -3.1444)
  line L651 (-35.1613, -3.1444) -> (-35.1613, -3.7108)
  line L652 (-35.1613, -3.7108) -> (-34.0016, -3.7108)
  line L653 (-34.0016, -3.7108) -> (-34.0016, -4.2821)
  line L654 (-34.0016, -4.2821) -> (-35.1613, -4.2821)
  line L655 (-35.1613, -4.2821) -> (-35.1613, -5.5731)
  line L656 (-35.1613, -5.5731) -> (-35.91, -5.5731)
  line L657 (-35.91, -5.5731) -> (-35.91, -2.5731)
  line L658 (-35.91, -2.5731) -> (-33.9019, -2.5731)
  line L659 (-33.9019, -2.5731) -> (-33.9019, -3.1444)
  line L660 (-32.3047, -5.5731) -> (-32.3047, -2.5731)
  line L661 (-32.3047, -2.5731) -> (-30.2771, -2.5731)
  line L662 (-30.2771, -2.5731) -> (-30.2771, -3.1444)
  line L663 (-30.2771, -3.1444) -> (-31.5559, -3.1444)
  line L664 (-31.5559, -3.1444) -> (-31.5559, -3.6719)
  line L665 (-31.5559, -3.6719) -> (-30.3768, -3.6719)
  line L666 (-30.3768, -3.6719) -> (-30.3768, -4.2432)
  line L667 (-30.3768, -4.2432) -> (-31.5559, -4.2432)
  line L668 (-31.5559, -4.2432) -> (-31.5559, -5.0018)
  line L669 (-31.5559, -5.0018) -> (-30.2771, -5.0018)
  line L670 (-30.2771, -5.0018) -> (-30.2771, -5.5731)
  line L671 (-30.2771, -5.5731) -> (-32.3047, -5.5731)
  line L672 (-27.1969, -5.5731) -> (-27.9214, -5.5731)
  line L673 (-27.9214, -5.5731) -> (-29.0786, -3.4823)
  line L674 (-29.0786, -3.4823) -> (-29.0786, -5.5731)
  line L675 (-29.0786, -5.5731) -> (-29.7666, -5.5731)
  line L676 (-29.7666, -5.5731) -> (-29.7666, -2.5731)
  line L677 (-29.7666, -2.5731) -> (-28.8428, -2.5731)
  line L678 (-28.8428, -2.5731) -> (-27.8849, -4.2919)
  line L679 (-27.8849, -4.2919) -> (-27.8849, -2.5731)
  line L680 (-27.8849, -2.5731) -> (-27.1969, -2.5731)
  line L681 (-27.1969, -2.5731) -> (-27.1969, -5.5731)
  spline S725 degree 2 poles (-24.0827, -5.4029) (-24.2796, -5.4831) (-24.9092, -5.6363) (-25.2156, -5.6363) knots 0 0 0 1 2 2 2
  spline S726 degree 2 poles (-25.2156, -5.6363) (-25.923, -5.6363) (-26.7617, -4.8194) (-26.7617, -4.0706) knots 0 0 0 1 2 2 2
  spline S727 degree 2 poles (-26.7617, -4.0706) (-26.7617, -3.3656) (-25.923, -2.5147) (-25.1937, -2.5147) knots 0 0 0 1 2 2 2
  spline S728 degree 2 poles (-25.1937, -2.5147) (-24.8169, -2.5147) (-24.3452, -2.6582) (-24.0948, -2.7797) knots 0 0 0 1 2 2 2
  line L682 (-24.0948, -2.7797) -> (-24.0948, -3.4847)
  line L683 (-24.0948, -3.4847) -> (-24.1629, -3.4847)
  spline S729 degree 2 poles (-24.1629, -3.4847) (-24.2164, -3.4434) (-24.4206, -3.2854) (-24.5178, -3.2319) knots 0 0 0 1 2 2 2
  spline S730 degree 2 poles (-24.5178, -3.2319) (-24.6297, -3.1663) (-24.9263, -3.0739) (-25.0916, -3.0739) knots 0 0 0 1 2 2 2
  spline S731 degree 2 poles (-25.0916, -3.0739) (-25.2836, -3.0739) (-25.6021, -3.1954) (-25.7261, -3.3194) knots 0 0 0 1 2 2 2
  spline S732 degree 2 poles (-25.7261, -3.3194) (-25.8452, -3.441) (-25.9838, -3.8129) (-25.9838, -4.0585) knots 0 0 0 1 2 2 2
  spline S733 degree 2 poles (-25.9838, -4.0585) (-25.9838, -4.5836) (-25.4562, -5.0844) (-25.0016, -5.0844) knots 0 0 0 1 2 2 2
  spline S734 degree 2 poles (-25.0016, -5.0844) (-24.9603, -5.0844) (-24.8533, -5.0796) (-24.812, -5.0771) knots 0 0 0 1 2 2 2
  line L684 (-24.812, -5.0771) -> (-24.812, -4.4864)
  line L685 (-24.812, -4.4864) -> (-25.393, -4.4864)
  line L686 (-25.393, -4.4864) -> (-25.393, -3.9248)
  line L687 (-25.393, -3.9248) -> (-24.0827, -3.9248)
  line L688 (-24.0827, -3.9248) -> (-24.0827, -5.4029)
  line L689 (-22.0211, -5.5731) -> (-23.6353, -5.5731)
  line L690 (-23.6353, -5.5731) -> (-23.6353, -5.0504)
  line L691 (-23.6353, -5.0504) -> (-23.205, -5.0504)
  line L692 (-23.205, -5.0504) -> (-23.205, -3.0958)
  line L693 (-23.205, -3.0958) -> (-23.6353, -3.0958)
  line L694 (-23.6353, -3.0958) -> (-23.6353, -2.5731)
  line L695 (-23.6353, -2.5731) -> (-22.0211, -2.5731)
  line L696 (-22.0211, -2.5731) -> (-22.0211, -3.0958)
  line L697 (-22.0211, -3.0958) -> (-22.4514, -3.0958)
  line L698 (-22.4514, -3.0958) -> (-22.4514, -5.0504)
  line L699 (-22.4514, -5.0504) -> (-22.0211, -5.0504)
  line L700 (-22.0211, -5.0504) -> (-22.0211, -5.5731)
  line L701 (-18.9506, -5.5731) -> (-19.675, -5.5731)
  line L702 (-19.675, -5.5731) -> (-20.8322, -3.4823)
  line L703 (-20.8322, -3.4823) -> (-20.8322, -5.5731)
  line L704 (-20.8322, -5.5731) -> (-21.5203, -5.5731)
  line L705 (-21.5203, -5.5731) -> (-21.5203, -2.5731)
  line L706 (-21.5203, -2.5731) -> (-20.5964, -2.5731)
  line L707 (-20.5964, -2.5731) -> (-19.6386, -4.2919)
  line L708 (-19.6386, -4.2919) -> (-19.6386, -2.5731)
  line L709 (-19.6386, -2.5731) -> (-18.9506, -2.5731)
  line L710 (-18.9506, -2.5731) -> (-18.9506, -5.5731)
  line L711 (-18.3404, -5.5731) -> (-18.3404, -2.5731)
  line L712 (-18.3404, -2.5731) -> (-16.3128, -2.5731)
  line L713 (-16.3128, -2.5731) -> (-16.3128, -3.1444)
  line L714 (-16.3128, -3.1444) -> (-17.5916, -3.1444)
  line L715 (-17.5916, -3.1444) -> (-17.5916, -3.6719)
  line L716 (-17.5916, -3.6719) -> (-16.4125, -3.6719)
  line L717 (-16.4125, -3.6719) -> (-16.4125, -4.2432)
  line L718 (-16.4125, -4.2432) -> (-17.5916, -4.2432)
  line L719 (-17.5916, -4.2432) -> (-17.5916, -5.0018)
  line L720 (-17.5916, -5.0018) -> (-16.3128, -5.0018)
  line L721 (-16.3128, -5.0018) -> (-16.3128, -5.5731)
  line L722 (-16.3128, -5.5731) -> (-18.3404, -5.5731)
  line L723 (-15.8023, -5.5731) -> (-15.8023, -2.5731)
  line L724 (-15.8023, -2.5731) -> (-13.7747, -2.5731)
  line L725 (-13.7747, -2.5731) -> (-13.7747, -3.1444)
  line L726 (-13.7747, -3.1444) -> (-15.0535, -3.1444)
  line L727 (-15.0535, -3.1444) -> (-15.0535, -3.6719)
  line L728 (-15.0535, -3.6719) -> (-13.8744, -3.6719)
  line L729 (-13.8744, -3.6719) -> (-13.8744, -4.2432)
  line L730 (-13.8744, -4.2432) -> (-15.0535, -4.2432)
  line L731 (-15.0535, -4.2432) -> (-15.0535, -5.0018)
  line L732 (-15.0535, -5.0018) -> (-13.7747, -5.0018)
  line L733 (-13.7747, -5.0018) -> (-13.7747, -5.5731)
  line L734 (-13.7747, -5.5731) -> (-15.8023, -5.5731)
  line L735 (-10.4927, -5.5731) -> (-11.4092, -5.5731)
  line L736 (-11.4092, -5.5731) -> (-12.2431, -4.4718)
  line L737 (-12.2431, -4.4718) -> (-12.5154, -4.4718)
  line L738 (-12.5154, -4.4718) -> (-12.5154, -5.5731)
  line L739 (-12.5154, -5.5731) -> (-13.2642, -5.5731)
  line L740 (-13.2642, -5.5731) -> (-13.2642, -2.5731)
  line L741 (-13.2642, -2.5731) -> (-12.0583, -2.5731)
  spline S735 degree 2 poles (-12.0583, -2.5731) (-11.8079, -2.5731) (-11.4384, -2.6363) (-11.2804, -2.7335) knots 0 0 0 1 2 2 2
  spline S736 degree 2 poles (-11.2804, -2.7335) (-11.1199, -2.8356) (-10.9303, -3.1541) (-10.9303, -3.3972) knots 0 0 0 1 2 2 2
  spline S737 degree 2 poles (-10.9303, -3.3972) (-10.9303, -3.74) (-11.2415, -4.1703) (-11.5016, -4.2967) knots 0 0 0 1 2 2 2
  line L742 (-11.5016, -4.2967) -> (-10.4927, -5.5731)
  spline S738 degree 2 poles (-11.7034, -3.492) (-11.7034, -3.3778) (-11.7909, -3.2149) (-11.8906, -3.1711) knots 0 0 0 1 2 2 2
  spline S739 degree 2 poles (-11.8906, -3.1711) (-11.9611, -3.1419) (-12.1337, -3.1249) (-12.2626, -3.1249) knots 0 0 0 1 2 2 2
  line L743 (-12.2626, -3.1249) -> (-12.5154, -3.1249)
  line L744 (-12.5154, -3.1249) -> (-12.5154, -3.9321)
  line L745 (-12.5154, -3.9321) -> (-12.299, -3.9321)
  spline S740 degree 2 poles (-12.299, -3.9321) (-12.1434, -3.9321) (-11.9222, -3.8932) (-11.8468, -3.8324) knots 0 0 0 1 2 2 2
  spline S741 degree 2 poles (-11.8468, -3.8324) (-11.7739, -3.774) (-11.7034, -3.6184) (-11.7034, -3.492) knots 0 0 0 1 2 2 2
  line L746 (-8.7763, -5.5731) -> (-10.3906, -5.5731)
  line L747 (-10.3906, -5.5731) -> (-10.3906, -5.0504)
  line L748 (-10.3906, -5.0504) -> (-9.9603, -5.0504)
  line L749 (-9.9603, -5.0504) -> (-9.9603, -3.0958)
  line L750 (-9.9603, -3.0958) -> (-10.3906, -3.0958)
  line L751 (-10.3906, -3.0958) -> (-10.3906, -2.5731)
  line L752 (-10.3906, -2.5731) -> (-8.7763, -2.5731)
  line L753 (-8.7763, -2.5731) -> (-8.7763, -3.0958)
  line L754 (-8.7763, -3.0958) -> (-9.2066, -3.0958)
  line L755 (-9.2066, -3.0958) -> (-9.2066, -5.0504)
  line L756 (-9.2066, -5.0504) -> (-8.7763, -5.0504)
  line L757 (-8.7763, -5.0504) -> (-8.7763, -5.5731)
  line L758 (-5.7058, -5.5731) -> (-6.4303, -5.5731)
  line L759 (-6.4303, -5.5731) -> (-7.5875, -3.4823)
  line L760 (-7.5875, -3.4823) -> (-7.5875, -5.5731)
  line L761 (-7.5875, -5.5731) -> (-8.2755, -5.5731)
  line L762 (-8.2755, -5.5731) -> (-8.2755, -2.5731)
  line L763 (-8.2755, -2.5731) -> (-7.3517, -2.5731)
  line L764 (-7.3517, -2.5731) -> (-6.3938, -4.2919)
  line L765 (-6.3938, -4.2919) -> (-6.3938, -2.5731)
  line L766 (-6.3938, -2.5731) -> (-5.7058, -2.5731)
  line L767 (-5.7058, -2.5731) -> (-5.7058, -5.5731)
  spline S742 degree 2 poles (-2.5916, -5.4029) (-2.7885, -5.4831) (-3.4181, -5.6363) (-3.7245, -5.6363) knots 0 0 0 1 2 2 2
  spline S743 degree 2 poles (-3.7245, -5.6363) (-4.4319, -5.6363) (-5.2707, -4.8194) (-5.2707, -4.0706) knots 0 0 0 1 2 2 2
  spline S744 degree 2 poles (-5.2707, -4.0706) (-5.2707, -3.3656) (-4.4319, -2.5147) (-3.7026, -2.5147) knots 0 0 0 1 2 2 2
  spline S745 degree 2 poles (-3.7026, -2.5147) (-3.3258, -2.5147) (-2.8541, -2.6582) (-2.6037, -2.7797) knots 0 0 0 1 2 2 2
  line L768 (-2.6037, -2.7797) -> (-2.6037, -3.4847)
  line L769 (-2.6037, -3.4847) -> (-2.6718, -3.4847)
  spline S746 degree 2 poles (-2.6718, -3.4847) (-2.7253, -3.4434) (-2.9295, -3.2854) (-3.0267, -3.2319) knots 0 0 0 1 2 2 2
  spline S747 degree 2 poles (-3.0267, -3.2319) (-3.1386, -3.1663) (-3.4352, -3.0739) (-3.6005, -3.0739) knots 0 0 0 1 2 2 2
  spline S748 degree 2 poles (-3.6005, -3.0739) (-3.7925, -3.0739) (-4.111, -3.1954) (-4.235, -3.3194) knots 0 0 0 1 2 2 2
  spline S749 degree 2 poles (-4.235, -3.3194) (-4.3541, -3.441) (-4.4927, -3.8129) (-4.4927, -4.0585) knots 0 0 0 1 2 2 2
  spline S750 degree 2 poles (-4.4927, -4.0585) (-4.4927, -4.5836) (-3.9652, -5.0844) (-3.5105, -5.0844) knots 0 0 0 1 2 2 2
  spline S751 degree 2 poles (-3.5105, -5.0844) (-3.4692, -5.0844) (-3.3622, -5.0796) (-3.3209, -5.0771) knots 0 0 0 1 2 2 2
  line L770 (-3.3209, -5.0771) -> (-3.3209, -4.4864)
  line L771 (-3.3209, -4.4864) -> (-3.9019, -4.4864)
  line L772 (-3.9019, -4.4864) -> (-3.9019, -3.9248)
  line L773 (-3.9019, -3.9248) -> (-2.5916, -3.9248)
  line L774 (-2.5916, -3.9248) -> (-2.5916, -5.4029)
  line L775 (-95.7885, -11.3415) -> (-96.5276, -11.3415)
  spline S752 degree 2 poles (-96.5276, -11.3415) (-96.6977, -11.1373) (-96.9773, -10.707) (-97.077, -10.459) knots 0 0 0 1 2 2 2
  spline S753 degree 2 poles (-97.077, -10.459) (-97.1718, -10.228) (-97.2788, -9.664) (-97.2788, -9.3601) knots 0 0 0 1 2 2 2
  spline S754 degree 2 poles (-97.2788, -9.3601) (-97.2788, -9.0271) (-97.1669, -8.4874) (-97.0794, -8.2637) knots 0 0 0 1 2 2 2
  spline S755 degree 2 poles (-97.0794, -8.2637) (-96.9822, -8.0206) (-96.7026, -7.5879) (-96.5276, -7.3788) knots 0 0 0 1 2 2 2
  line L776 (-96.5276, -7.3788) -> (-95.7885, -7.3788)
  line L777 (-95.7885, -7.3788) -> (-95.7885, -7.4371)
  spline S756 degree 2 poles (-95.7885, -7.4371) (-95.9514, -7.583) (-96.248, -7.9574) (-96.3744, -8.2054) knots 0 0 0 1 2 2 2
  spline S757 degree 2 poles (-96.3744, -8.2054) (-96.4959, -8.446) (-96.6467, -9.0295) (-96.6467, -9.3601) knots 0 0 0 1 2 2 2
  spline S758 degree 2 poles (-96.6467, -9.3601) (-96.6467, -9.7054) (-96.5008, -10.2645) (-96.3744, -10.5149) knots 0 0 0 1 2 2 2
  spline S759 degree 2 poles (-96.3744, -10.5149) (-96.2528, -10.7507) (-95.9489, -11.1397) (-95.7885, -11.2832) knots 0 0 0 1 2 2 2
  line L778 (-95.7885, -11.2832) -> (-95.7885, -11.3415)
  line L779 (-92.2512, -10.5125) -> (-93, -10.5125)
  line L780 (-93, -10.5125) -> (-93, -8.5238)
  line L781 (-93, -8.5238) -> (-93.5446, -9.8075)
  line L782 (-93.5446, -9.8075) -> (-94.06, -9.8075)
  line L783 (-94.06, -9.8075) -> (-94.6045, -8.5238)
  line L784 (-94.6045, -8.5238) -> (-94.6045, -10.5125)
  line L785 (-94.6045, -10.5125) -> (-95.3144, -10.5125)
  line L786 (-95.3144, -10.5125) -> (-95.3144, -7.5125)
  line L787 (-95.3144, -7.5125) -> (-94.4465, -7.5125)
  line L788 (-94.4465, -7.5125) -> (-93.7804, -8.993)
  line L789 (-93.7804, -8.993) -> (-93.1191, -7.5125)
  line L790 (-93.1191, -7.5125) -> (-92.2512, -7.5125)
  line L791 (-92.2512, -7.5125) -> (-92.2512, -10.5125)
  spline S760 degree 2 poles (-90.5105, -10.5733) (-91.1523, -10.5733) (-91.8355, -9.9606) (-91.8355, -9.3942) knots 0 0 0 1 2 2 2
  spline S761 degree 2 poles (-91.8355, -9.3942) (-91.8355, -8.8399) (-91.1985, -8.1786) (-90.6248, -8.1786) knots 0 0 0 1 2 2 2
  spline S762 degree 2 poles (-90.6248, -8.1786) (-90.107, -8.1786) (-89.5818, -8.7402) (-89.5818, -9.2605) knots 0 0 0 1 2 2 2
  line L792 (-89.5818, -9.2605) -> (-89.5818, -9.5157)
  line L793 (-89.5818, -9.5157) -> (-91.1305, -9.5157)
  spline S763 degree 2 poles (-91.1305, -9.5157) (-91.1207, -9.6738) (-91.0065, -9.8828) (-90.9141, -9.946) knots 0 0 0 1 2 2 2
  spline S764 degree 2 poles (-90.9141, -9.946) (-90.8241, -10.0092) (-90.581, -10.0627) (-90.4376, -10.0627) knots 0 0 0 1 2 2 2
  spline S765 degree 2 poles (-90.4376, -10.0627) (-90.316, -10.0627) (-90.0778, -10.0092) (-89.9781, -9.9631) knots 0 0 0 1 2 2 2
  spline S766 degree 2 poles (-89.9781, -9.9631) (-89.8906, -9.9266) (-89.7447, -9.8366) (-89.6985, -9.8026) knots 0 0 0 1 2 2 2
  line L794 (-89.6985, -9.8026) -> (-89.6232, -9.8026)
  line L795 (-89.6232, -9.8026) -> (-89.6232, -10.3861)
  spline S767 degree 2 poles (-89.6232, -10.3861) (-89.7107, -10.4201) (-89.8517, -10.4785) (-89.9781, -10.5076) knots 0 0 0 1 2 2 2
  spline S768 degree 2 poles (-89.9781, -10.5076) (-90.0924, -10.5392) (-90.3355, -10.5733) (-90.5105, -10.5733) knots 0 0 0 1 2 2 2
  spline S769 degree 2 poles (-90.2771, -9.0903) (-90.282, -8.8666) (-90.4789, -8.6308) (-90.6807, -8.6308) knots 0 0 0 1 2 2 2
  spline S770 degree 2 poles (-90.6807, -8.6308) (-90.8874, -8.6308) (-91.1207, -8.8788) (-91.1329, -9.0903) knots 0 0 0 1 2 2 2
  line L796 (-91.1329, -9.0903) -> (-90.2771, -9.0903)
  spline S771 degree 2 poles (-88.111, -10.5733) (-88.3906, -10.5733) (-88.8549, -10.4323) (-89.0276, -10.2864) knots 0 0 0 1 2 2 2
  spline S772 degree 2 poles (-89.0276, -10.2864) (-89.1953, -10.1381) (-89.3849, -9.6932) (-89.3849, -9.3917) knots 0 0 0 1 2 2 2
  spline S773 degree 2 poles (-89.3849, -9.3917) (-89.3849, -9.066) (-89.1807, -8.6114) (-89.0032, -8.4655) knots 0 0 0 1 2 2 2
  spline S774 degree 2 poles (-89.0032, -8.4655) (-88.8355, -8.3245) (-88.3784, -8.1883) (-88.1305, -8.1883) knots 0 0 0 1 2 2 2
  spline S775 degree 2 poles (-88.1305, -8.1883) (-87.9433, -8.1883) (-87.5689, -8.2759) (-87.3793, -8.3707) knots 0 0 0 1 2 2 2
  line L797 (-87.3793, -8.3707) -> (-87.3793, -8.9736)
  line L798 (-87.3793, -8.9736) -> (-87.4692, -8.9736)
  spline S776 degree 2 poles (-87.4692, -8.9736) (-87.513, -8.9323) (-87.6345, -8.835) (-87.7075, -8.7961) knots 0 0 0 1 2 2 2
  spline S777 degree 2 poles (-87.7075, -8.7961) (-87.7853, -8.7524) (-87.9773, -8.694) (-88.0964, -8.694) knots 0 0 0 1 2 2 2
  spline S778 degree 2 poles (-88.0964, -8.694) (-88.3663, -8.694) (-88.6629, -9.0708) (-88.6629, -9.3917) knots 0 0 0 1 2 2 2
  spline S779 degree 2 poles (-88.6629, -9.3917) (-88.6629, -9.7321) (-88.3468, -10.0676) (-88.0843, -10.0676) knots 0 0 0 1 2 2 2
  spline S780 degree 2 poles (-88.0843, -10.0676) (-87.9506, -10.0676) (-87.7512, -10.0068) (-87.6783, -9.9631) knots 0 0 0 1 2 2 2
  spline S781 degree 2 poles (-87.6783, -9.9631) (-87.6078, -9.9217) (-87.5057, -9.8293) (-87.4692, -9.7929) knots 0 0 0 1 2 2 2
  line L799 (-87.4692, -9.7929) -> (-87.3793, -9.7929)
  line L800 (-87.3793, -9.7929) -> (-87.3793, -10.3982)
  spline S782 degree 2 poles (-87.3793, -10.3982) (-87.44, -10.425) (-87.5981, -10.493) (-87.6807, -10.5149) knots 0 0 0 1 2 2 2
  spline S783 degree 2 poles (-87.6807, -10.5149) (-87.7828, -10.5441) (-87.9627, -10.5733) (-88.111, -10.5733) knots 0 0 0 1 2 2 2
  line L801 (-84.9263, -10.5125) -> (-85.6361, -10.5125)
  line L802 (-85.6361, -10.5125) -> (-85.6361, -9.3917)
  spline S784 degree 2 poles (-85.6361, -9.3917) (-85.6361, -9.2532) (-85.658, -8.9809) (-85.6872, -8.9177) knots 0 0 0 1 2 2 2
  spline S785 degree 2 poles (-85.6872, -8.9177) (-85.7237, -8.8399) (-85.8598, -8.7742) (-85.9765, -8.7742) knots 0 0 0 1 2 2 2
  spline S786 degree 2 poles (-85.9765, -8.7742) (-86.0616, -8.7742) (-86.2391, -8.8399) (-86.3387, -8.9104) knots 0 0 0 1 2 2 2
  line L803 (-86.3387, -8.9104) -> (-86.3387, -10.5125)
  line L804 (-86.3387, -10.5125) -> (-87.0438, -10.5125)
  line L805 (-87.0438, -10.5125) -> (-87.0438, -7.3788)
  line L806 (-87.0438, -7.3788) -> (-86.3387, -7.3788)
  line L807 (-86.3387, -7.3788) -> (-86.3387, -8.4995)
  spline S787 degree 2 poles (-86.3387, -8.4995) (-86.1661, -8.3537) (-85.8379, -8.1883) (-85.6386, -8.1883) knots 0 0 0 1 2 2 2
  spline S788 degree 2 poles (-85.6386, -8.1883) (-85.2934, -8.1883) (-84.9263, -8.6259) (-84.9263, -9.0392) knots 0 0 0 1 2 2 2
  line L808 (-84.9263, -9.0392) -> (-84.9263, -10.5125)
  spline S789 degree 2 poles (-83.1564, -10.2718) (-83.2293, -10.3326) (-83.3436, -10.4298) (-83.4408, -10.4785) knots 0 0 0 1 2 2 2
  spline S790 degree 2 poles (-83.4408, -10.4785) (-83.5357, -10.5246) (-83.7156, -10.5733) (-83.876, -10.5733) knots 0 0 0 1 2 2 2